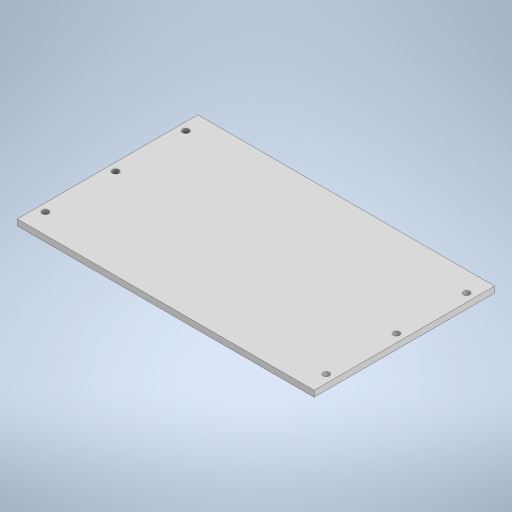
# Autodesk Inventor part: chest_cover_top
Saved by Autodesk Inventor 2024.1 (Build 281209000, 209)
## iProperties
Created: 2024-02-14
Part Number: chest_cover_top
Material: 一般
Document SubType Name: Modeling
Designer: hibik
Density: 1 g/cm^3
Appearance: 既定
Author: hibik
Autodesk Inventor part; units mm, degrees
ref_plane "YZ Plane" through (0, 0, 0) normal (1, 0, 0) x (0, 1, 0)
ref_plane "XZ Plane" through (0, 0, 0) normal (0, 1, 0) x (-1, 0, 0)
ref_plane "XY Plane" through (0, 0, 0) normal (0, 0, 1) x (1, 0, 0)
sketch "スケッチ1" plane through (0, 0, 0) normal (0, 1, 0) x (-1, 0, 0)
  line L0 (30, 0) -> (-30, 0)
  line L1 (-30, 0) -> (-30, -45)
  line L2 (-30, -45) -> (30, -45)
  line L3 (30, -45) -> (30, 0)
  line L4 (37, 0) -> (30, 0)
  line L5 (30, 0) -> (30, -45)
  line L6 (30, -45) -> (37, -45)
  line L7 (37, -45) -> (37, 0)
  line L8 (-30, 0) -> (-37, 0)
  line L9 (-37, 0) -> (-37, -45)
  line L10 (-37, -45) -> (-30, -45)
  line L11 (-30, -45) -> (-30, 0)
  line L12 (37, 0) -> (35, 0)
  line L13 (35, 0) -> (35, -45) construction
  line L14 (35, -45) -> (37, -45)
  line L15 (37, -45) -> (37, 0)
  line L16 (-37, 0) -> (-35, 0)
  line L17 (-35, 0) -> (-35, -45) construction
  line L18 (-35, -45) -> (-37, -45)
  line L19 (-37, -45) -> (-37, 0)
  circle A0 centre (35, -5) radius 0.8
  circle A1 centre (35, -40) radius 0.8
  circle A2 centre (-35, -5) radius 0.8
  circle A3 centre (-35, -40) radius 0.8
  circle A4 centre (-35, -22.5) radius 0.8
  circle A5 centre (35, -22.5) radius 0.8
  point P0 (0, 0)
  point P1 (0, 0)
  point P2 (30, 0)
  dimension "d0" = 60
  dimension "d1" = 45
  dimension "d4" = 7
  dimension "d5" = 2
  dimension "d6" = 2
  dimension "d7" = 1.6
  dimension "d8" = 1.6
  dimension "d9" = 1.6
  dimension "d10" = 1.6
  dimension "d11" = 5
  dimension "d12" = 5
  dimension "d13" = 1.6
  dimension "d14" = 1.6
  constraints: 40 end point, 10 parallel, 6 centre point, 6 point on line, 5 horizontal, 5 perpendicular, 3 collinear, 3 midpoint, 2 horizontal alignment, 1 coincident
  measures "d0" distance of L0.start L0.end
  measures "d1" distance of L2.end L0.start
  measures "d4" distance of L4.start L4.end
  measures "d5" distance between parallel lines of L15 L13
  measures "d6" distance between parallel lines of L19 L17
  measures "d7" diameter of A0
  measures "d8" diameter of A1
  measures "d9" diameter of A2
  measures "d10" diameter of A3
  measures "d11" distance from line of L8 A2.centre
  measures "d12" distance from line of L10 A3.centre
  measures "d13" diameter of A4
  measures "d14" diameter of A5
extrude "押し出し1" add sketch "スケッチ1" along normal blind 1.5
